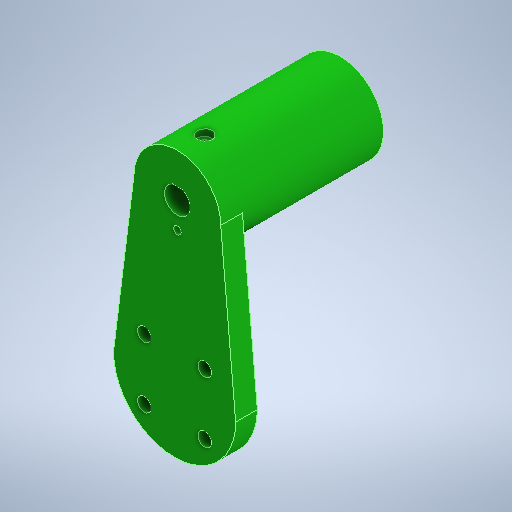
# Autodesk Inventor part: pen_holder
Saved by Autodesk Inventor 2025.1 (Build 291241000, 241)
## iProperties
Created: 2024-08-22
Part Number: pen_holder
Material: LCP Plastic
Document SubType Name: Modeling
Designer: pedro
Density: 1.626 g/cm^3
Appearance: Dark Green
Author: pedro
Autodesk Inventor part; units mm, degrees
ref_plane "YZ Plane" through (0, 0, 0) normal (1, 0, 0) x (0, 1, 0)
ref_plane "XZ Plane" through (0, 0, 0) normal (0, 1, 0) x (-1, 0, 0)
sketch "Sketch1" plane through (0, 0, 0) normal (0, 0, 1) x (1, 0, 0)
  arc A0 (-22.5, 0) -> (22.5, 0) centre (0, 0) ccw
  circle A1 centre (-11.1871, 11.1871) radius 2.5
  arc A2 (17, 60) -> (-15, 60) centre (1, 60) ccw
  line L0 (22.5, 0) -> (17, 60)
  line L1 (-22.5, 0) -> (-15, 60)
  circle A3 centre (11.0869, 11.1871) radius 2.5
  line L2 (-1.4379, 0) -> (3.0127, 0) construction
  circle A4 centre (-11.1871, -11.1871) radius 2.5
  circle A5 centre (11.0869, -11.1871) radius 2.5
  dimension "d0" = 45
  dimension "d3" = 5
  dimension "d29" = 32
  dimension "d57" = 5
  dimension "d58" = 22.274
  dimension "d59" = 15.821
  constraints: 6 centre point, 6 end point, 4 point on circle, 2 symmetric about line, 1 coincident, 1 horizontal, 2 other
  measures "d0" diameter of A0
  measures "d3" diameter of A1
  measures "d29" diameter of A2
  measures "d57" diameter of A3
  measures "d58" distance of A3.centre A1.centre
  measures "d59" distance of point (0, 0) A1.centre
extrude "Extrusion1" add sketch "Sketch1" along normal blind 8
sketch "Sketch5" plane through (0, 0, 8) normal (0, 0, 1) x (1, 0, 0)
  arc A0 (17, 60) -> (-15, 60) centre (1, 60) ccw projected
  circle A1 centre (1, 60) radius 16
  point P0 (0, 0)
  point P1 (-15, 60)
  dimension "d44" = 32
  constraints: 1 centre point, 1 coincident
  measures "d44" diameter of A1
extrude "Extrusion3" add sketch "Sketch5" against normal blind 60
sketch "Sketch6" plane through (0, 0, 8) normal (0, 0, 1) x (1, 0, 0)
  arc A0 (17, 60) -> (-15, 60) centre (1, 60) ccw projected
  arc A1 (-0.9268, 64.2869) -> (2.9268, 64.2869) centre (1, 60) ccw
  line L0 (-0.9268, 64.2869) -> (2.9268, 64.2869)
  point P0 (0, 0)
  point P1 (1, 55.3)
  point P2 (1, 64.2869)
  dimension "d32" = 9.4
  dimension "d43" = 4.2869
  constraints: 3 point on circle, 2 end point, 1 centre point, 1 coincident, 1 horizontal, 1 midpoint
  measures "d32" diameter of A1
  measures "d43" distance of A1.centre point (1, 64.287)
extrude "Extrusion4" cut sketch "Sketch6" against normal through all
ref_plane "Work Plane2" through (1, 76, 8) normal (0, 1, 0) x (-1, 0, 0)
sketch "Sketch9" plane through (1, 76, 8) normal (0, 1, 0) x (-1, 0, 0)
  line L0 (16, 0) -> (-16, 0) projected
  line L1 (0, 0) -> (0, -10)
  circle A0 centre (0, -10) radius 1.35
  point P0 (1, -8)
  dimension "d45" = 10
  dimension "d46" = 2.7
  constraints: 2 end point, 1 centre point, 1 coincident, 1 midpoint, 1 vertical
  measures "d45" distance of L1.start L1.end
  measures "d46" diameter of A0
extrude "Extrusion7" cut sketch "Sketch9" against normal blind 12
sketch "Sketch10" plane through (1, 76, 8) normal (0, 1, 0) x (-1, 0, 0)
  circle A0 centre (0, -10) radius 1.35 projected
  circle A1 centre (0, -10) radius 2.75
  point P0 (1, -8)
  dimension "d49" = 5.5
  constraints: 1 centre point, 1 coincident
  measures "d49" diameter of A1
extrude "Extrusion8" cut sketch "Sketch10" against normal blind 2.5
sketch "Sketch13" plane through (0, 0, 8) normal (0, 0, 1) x (1, 0, 0)
  circle A0 centre (1, 50.438) radius 1.4
  arc A1 (-0.9268, 64.2869) -> (2.9268, 64.2869) centre (1, 60) ccw projected
  point P0 (0, 0)
  dimension "d60" = 2.8
  dimension "d61" = 9.562
  constraints: 1 centre point
  measures "d60" diameter of A0
  measures "d61" distance of A1.centre A0.centre
extrude "Extrusion11" cut sketch "Sketch13" against normal blind 15
body "Solid1"
